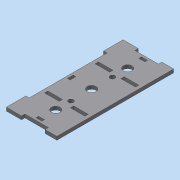
# Autodesk Inventor part: X-Anchor_Front-Inner
Saved by Autodesk Inventor 2016 SP1 (Build 200210100, 210)
## iProperties
Created: 2016-03-01
Part Number: X-Anchor_Front-Inner
Material: Generic
Document SubType Name: Modeling
Designer: Mohamed A.
Density: 1 g/cm^3
Appearance: Default
Author: Mohamed A.
Autodesk Inventor part; units mm, degrees
ref_plane "YZ Plane" through (0, 0, 0) normal (1, 0, 0) x (0, 1, 0)
ref_plane "XZ Plane" through (0, 0, 0) normal (0, 1, 0) x (-1, 0, 0)
ref_plane "XY Plane" through (0, 0, 0) normal (0, 0, 1) x (1, 0, 0)
sketch "Sketch1" plane through (0, 0, 0) normal (0, 0, 1) x (1, 0, 0)
  circle A0 centre (0, 0) radius 11 construction
  circle A1 centre (0, -32) radius 3.9 projected
  circle A2 centre (0, 32) radius 3.9 projected
  line L0 (-5, 21) -> (-5, 24) projected
  line L1 (-5, 24) -> (-18, 24) projected
  line L2 (-18, 24) -> (-18, 21) projected
  line L3 (-18, 21) -> (-5, 21) projected
  line L4 (18, 21) -> (18, 24) projected
  line L5 (18, 24) -> (5, 24) projected
  line L6 (5, 24) -> (5, 21) projected
  line L7 (5, 21) -> (18, 21) projected
  line L8 (-5, -24) -> (-5, -21) projected
  line L9 (-5, -21) -> (-18, -21) projected
  line L10 (-18, -21) -> (-18, -24) projected
  line L11 (-18, -24) -> (-5, -24) projected
  line L12 (18, -24) -> (18, -21) projected
  line L13 (18, -21) -> (5, -21) projected
  line L14 (5, -21) -> (5, -24) projected
  line L15 (5, -24) -> (18, -24) projected
  line L16 (-19, -2.65) -> (-16.6, -2.65) projected
  line L17 (-16.6, -2.65) -> (-16.6, 2.65) projected
  line L18 (-16.6, 2.65) -> (-19, 2.65) projected
  line L19 (-19, 2.65) -> (-19, -2.65) projected
  line L20 (-2.65, -44.6) -> (-2.65, -47) projected
  line L21 (-2.65, -47) -> (2.65, -47) projected
  line L22 (2.65, -47) -> (2.65, -44.6) projected
  line L23 (2.65, -44.6) -> (-2.65, -44.6) projected
  line L24 (-2.65, 44.6) -> (2.65, 44.6) projected
  line L25 (2.65, 44.6) -> (2.65, 47) projected
  line L26 (2.65, 47) -> (-2.65, 47) projected
  line L27 (-2.65, 47) -> (-2.65, 44.6) projected
  circle A3 centre (15.5, 15.5) radius 1.4 projected
  circle A4 centre (-15.5, 15.5) radius 1.4 projected
  circle A5 centre (-15.5, -15.5) radius 1.4 projected
  circle A6 centre (15.5, -15.5) radius 1.4 projected
  line L28 (-10.5, -49) -> (-10.5, -52) projected
  line L29 (-10.5, -52) -> (-24, -52) projected
  line L30 (-24, -52) -> (-24, -34.6667) projected
  line L31 (-24, -34.6667) -> (-21, -34.6667) projected
  line L32 (-21, -34.6667) -> (-21, 34.6667) projected
  line L33 (-21, 34.6667) -> (-24, 34.6667) projected
  line L34 (-24, 34.6667) -> (-24, 52) projected
  line L35 (-24, 52) -> (-10.5, 52) projected
  line L36 (-10.5, 52) -> (-10.5, 49) projected
  line L37 (-10.5, 49) -> (10.5, 49) projected
  line L38 (10.5, 49) -> (10.5, 52) projected
  line L39 (10.5, 52) -> (21, 52) projected
  line L40 (21, 52) -> (21, -52) projected
  line L41 (21, -52) -> (10.5, -52) projected
  line L42 (10.5, -52) -> (10.5, -49) projected
  line L43 (10.5, -49) -> (-10.5, -49) projected
  circle A7 centre (0, 0) radius 4
  circle A8 centre (0, -18.5) radius 2.4 construction
  circle A9 centre (0, 18.5) radius 2.4 construction
  circle A10 centre (0, 18.5) radius 2.2
  circle A11 centre (0, -18.5) radius 2.2
  point P0 (0, 0)
  dimension "d2" = 8
  dimension "d3" = 0.2
  dimension "d4" = 0.2
  constraints: 3 centre point, 1 coincident
  measures "d2" diameter of A7
  measures "d3" radial gap between concentric circles of A9 A10
  measures "d4" radial gap between concentric circles of A8 A11
extrude "Extrusion1" add sketch "Sketch1" along normal blind 3 contours A3 | A4 | A5 | A6 | L28 L29 L30 L31 L32 L33 L34 L35 L36 L37 L38 L39 L40 L41 L42 L43
body "Solid1"
